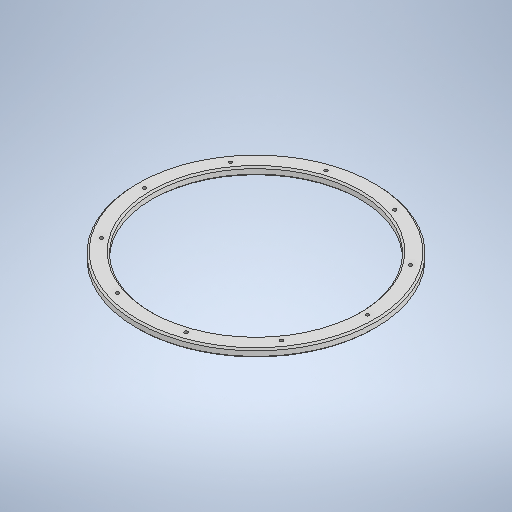
# Autodesk Inventor part: Pieza3
Saved by Autodesk Inventor 2025.1 (Build 291241000, 241)
## iProperties
Created: 2024-10-07
Part Number: Pieza3
Material: Genérico
Document SubType Name: Sheet Metal
Designer: Octavio
Density: 1 g/cm^3
Sheet Metal Rule: Por defecto_mm
Appearance: Valor por defecto
Author: Octavio
Autodesk Inventor part; units mm, degrees
ref_plane "YZ Plane" through (0, 0, 0) normal (1, 0, 0) x (0, 1, 0)
ref_plane "XZ Plane" through (0, 0, 0) normal (0, 1, 0) x (-1, 0, 0)
ref_plane "XY Plane" through (0, 0, 0) normal (0, 0, 1) x (1, 0, 0)
sketch "Boceto1" plane through (0, 0, 0) normal (0, 0, 1) x (1, 0, 0)
  line L0 (-150, 4.9659) -> (-130, 4.9659)
  line L1 (-130, 4.9659) -> (-130, -5.0341)
  line L2 (-130, -5.0341) -> (-150, -5.0341)
  line L3 (-150, -5.0341) -> (-150, 4.9659)
  line L4 (0, 0) -> (0, 54.3262)
  dimension "d0" = 20
  dimension "d1" = 10
  dimension "d2" = 150
  constraints: 10 end point, 2 parallel, 1 horizontal, 1 perpendicular, 1 vertical
  measures "d0" distance of L1.end L2.end
  measures "d1" distance of L0.end L1.end
  measures "d2" distance from line of L3 L4.start
revolve "Revolución1" add sketch "Boceto1" angle 360 about axis through (0, 0, 0) along (0, 1, 0)
chamfer "Chaflán1" distance 2 angle 45 4 edges at (150, 4.9659, 0) (130, 4.9659, 0) (150, -5.0341, 0) (130, -5.0341, 0)
sketch "Boceto2" plane through (0, 4.9659, 0) normal (0, 1, 0) x (1, 0, 0)
  point P0 (0, 0)
  point P1 (-138.7138, -0.9769)
hole "Agujero1" at (-138.7138, 4.9659, 0.9769) direction (0, -1, 0) diameter 4.134 end through all thread size "M5x0.8" class "6H" standard "ISO Metric profile"
pattern_circular "Patrón circular1" count 10 over 360 about axis through (0, -10, 0) along (0, 1, 0) of "Agujero1"
equation "\"d12\" = Grosor"
equation "\"Radio_pliegue\" = Grosor"
equation "\"Anchura_desahogo_plegado\" = Grosor"
equation "\"Profundidad_desahogo_plegado\" = 0.5 * Grosor"
equation "\"Tamaño_destalonado\" = 4 * Grosor"
equation "\"Remanente_mínimo\" = 2 * Grosor"
equation "\"Radiodetransición\" = Radio_pliegue"
equation "\"Tamaño_de_radio_de_Jacobi\" = Radio_pliegue"
equation "\"TamañoSeparación\" = Grosor"
equation "\"Grosor\" = 0.5"
